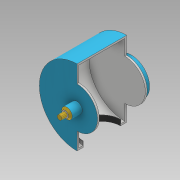
# Autodesk Inventor part: 헤드(상)
Saved by Autodesk Inventor 2018 (Build 220112000, 112)
## iProperties
Created: 2018-04-19
Part Number: 헤드(상)
Material: 일반
Document SubType Name: Modeling
Designer: CK
Density: 1 g/cm^3
Appearance: 기본값
Mass: 32.7883 g
Surface Area: 274.058 cm^2
Volume: 32.7883 cm^3
Author: CK
Autodesk Inventor part; units mm, degrees
ref_plane "YZ Plane" through (0, 0, 0) normal (1, 0, 0) x (0, 1, 0)
ref_plane "XZ Plane" through (0, 0, 0) normal (0, 1, 0) x (-1, 0, 0)
sketch "스케치1" plane through (0, 0, 0) normal (0, 1, 0) x (-1, 0, 0)
  arc A0 (0, -41) -> (0, 41) centre (0, 0) ccw
  line L0 (0, 41) -> (0, -41)
  dimension "d0" = 82
  constraints: 2 end point, 2 point on circle, 1 centre point, 1 coincident, 1 vertical
  measures "d0" diameter of A0
extrude "돌출1" add sketch "스케치1" along normal mid plane 54
shell "쉘1" thickness 2 removed faces 1 at (0, 9, -13.6667)
sketch "스케치3" plane through (0, 27, 0) normal (0, 1, 0) x (1, 0, 0)
  circle A0 centre (0, 0) radius 22.25
  line L0 (0, 41) -> (0, -41) projected
  line L1 (0, -22.25) -> (0, 22.25)
  dimension "d4" = 44.5
  constraints: 2 end point, 2 point on circle, 2 point on line, 1 centre point, 1 coincident
  measures "d4" diameter of A0
extrude "돌출2" add sketch "스케치3" against normal blind 2 contours A0 L0 picked at (7.4489, 4.8102)
mirror "미러1" about plane through (0, 0, 0) normal (0, 1, 0) of "돌출2"
sketch "스케치4" plane through (0, 27, 0) normal (0, 1, 0) x (1, 0, 0)
  circle A0 centre (0, 0) radius 20
  dimension "d7" = 40
  constraints: 1 centre point, 1 coincident
  measures "d7" diameter of A0
extrude "돌출3" add sketch "스케치4" along normal blind 5
sketch "스케치5" plane through (0, 32, 0) normal (0, 1, 0) x (1, 0, 0)
  circle A0 centre (0, 0) radius 2.5
  dimension "d10" = 5
  constraints: 1 centre point, 1 coincident
  measures "d10" diameter of A0
extrude "돌출4" add sketch "스케치5" along normal blind 7
sketch "스케치6" plane through (0, -27, 0) normal (0, -1, 0) x (1, 0, 0)
  circle A0 centre (0, 0) radius 5.75
  dimension "d13" = 11.5
  constraints: 1 centre point, 1 coincident
  measures "d13" diameter of A0
extrude "돌출5" add sketch "스케치6" along normal blind 13
sketch "스케치7" plane through (0, -40, 0) normal (0, -1, 0) x (1, 0, 0)
  circle A0 centre (0, 0) radius 2.5
  dimension "d16" = 5
  constraints: 1 centre point, 1 coincident
  measures "d16" diameter of A0
extrude "돌출6" add sketch "스케치7" along normal blind 6
chamfer "모따기1" distance 2 angle 45 1 edges at (-5.75, -40, 0)
ref_plane "작업 평면1" through (0, 0, -41) normal (0, 0, 1) x (1, 0, 0)
sketch "스케치8" plane through (0, 0, -41) normal (0, 0, 1) x (1, 0, 0)
  circle A0 centre (0, 0) radius 20.5
  dimension "d23" = 41
  constraints: 1 centre point, 1 coincident
  measures "d23" diameter of A0
extrude "돌출7" cut sketch "스케치8" along normal up to surface round surface about axis through (0, 0, 0) along (0, 1, 0) radius 39 far side no
ref_plane "작업 평면2" through (0, 0, -41) normal (0, 0, 1) x (1, 0, 0)
sketch "스케치9" plane through (0, 0, -41) normal (0, 0, 1) x (1, 0, 0)
  circle A0 centre (0, 0) radius 20.5
  line L0 (0, 25) -> (0, 20.5) projected
  line L1 (0, 20.5) -> (0, -20.5)
  dimension "d27" = 41
  constraints: 2 end point, 1 centre point, 1 coincident, 1 collinear, 1 point on circle
  measures "d27" diameter of A0
extrude "돌출8" add sketch "스케치9" along normal blind 6 contours L1 A0 picked at (-6.7835, -0.8237)
sketch "스케치10" plane through (0, 0, -41) normal (0, 0, -1) x (-1, 0, 0)
  circle A0 centre (0, 0) radius 20.25
  dimension "d30" = 40.5
  constraints: 1 centre point, 1 coincident
  measures "d30" diameter of A0
extrude "돌출9" cut sketch "스케치10" against normal blind 10
